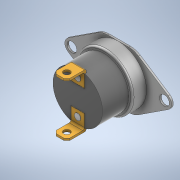
# Autodesk Inventor part: Bimetallschalter
Saved by Autodesk Inventor 2021 (Build 250183000, 183)
## iProperties
Created: 2021-04-29
Part Number: Bimetallschalter
Material: Generisch
Document SubType Name: Modeling
Designer: Sebastian Seewald
Density: 1 g/cm^3
Appearance: Vorgabe
Author: Sebastian Seewald
Autodesk Inventor part; units mm, degrees
ref_plane "YZ Plane" through (0, 0, 0) normal (1, 0, 0) x (0, 1, 0)
ref_plane "XZ Plane" through (0, 0, 0) normal (0, 1, 0) x (-1, 0, 0)
ref_plane "XY Plane" through (0, 0, 0) normal (0, 0, 1) x (1, 0, 0)
sketch "Skizze1" plane through (0, 0, 0) normal (0, 0, 1) x (1, 0, 0)
  line L0 (-3, 8) -> (3, 8)
  line L1 (5.7352, 7.1856) -> (14.1691, 1.6742)
  line L2 (14.1691, -1.6742) -> (5.7352, -7.1856)
  line L3 (3, -8) -> (-3, -8)
  line L4 (-5.7352, -7.1856) -> (-14.1691, -1.6742)
  line L5 (-14.1691, 1.6742) -> (-5.7352, 7.1856)
  arc A0 (14.1691, -1.6742) -> (14.1691, 1.6742) centre (13.075, 0) ccw
  arc A1 (-14.1691, 1.6742) -> (-14.1691, -1.6742) centre (-13.075, 0) ccw
  circle A2 centre (0, 0) radius 7
  circle A3 centre (-13.075, 0) radius 1.385
  circle A4 centre (13.075, 0) radius 1.385
  arc A5 (-3, 8) -> (-5.7352, 7.1856) centre (-3, 3) ccw
  arc A6 (5.7352, 7.1856) -> (3, 8) centre (3, 3) ccw
  arc A7 (3, -8) -> (5.7352, -7.1856) centre (3, -3) ccw
  arc A8 (-5.7352, -7.1856) -> (-3, -8) centre (-3, -3) ccw
  dimension "d0" = 16
  dimension "d1" = 8
  dimension "d3" = 2
  dimension "d4" = 14
  dimension "d5" = 30.15
  dimension "d7" = 2.77
  dimension "d8" = 2.77
  dimension "d9" = 13.075
  dimension "d10" = 13.075
  dimension "d11" = 5
  dimension "d12" = 6
  dimension "d13" = 6
  dimension "d14" = 3
  dimension "d15" = 3
  constraints: 12 end point, 12 point on circle, 12 tangent, 9 centre point, 4 equal radius, 3 coincident, 1 horizontal, 1 horizontal alignment, 1 parallel
  measures "d0" distance between parallel lines of L3 L0
  measures "d1" distance from line of point (0, 0) L0
  measures "d3" radius of A0
  measures "d4" diameter of A2
  measures "d7" diameter of A3
  measures "d8" diameter of A4
  measures "d9" distance of A1.centre point (0, 0)
  measures "d10" distance of A0.centre point (0, 0)
  measures "d11" radius of A5
  measures "d12" distance of L0.start L0.end
  measures "d13" distance of L3.start L3.end
  measures "d14" horizontal distance of point (0, 0) L0.start
  measures "d15" horizontal distance of point (0, 0) L3.end
extrude "Extrusion1" add sketch "Skizze1" along normal blind 0.5
sketch "Skizze2" plane through (0, 0, 0.5) normal (0, 0, 1) x (1, 0, 0)
  circle A0 centre (0, 0) radius 8
  circle A1 centre (0, 0) radius 7
  dimension "d18" = 16
  dimension "d19" = 14
  constraints: 2 centre point, 2 coincident
  measures "d18" diameter of A0
  measures "d19" diameter of A1
extrude "Extrusion2" add sketch "Skizze2" along normal blind 4
fillet "Rundung1" radius 0.5 1 edges at (-8, 0, 4.5)
sketch "Skizze3" plane through (0, 0, 0) normal (0, 0, -1) x (-1, 0, 0)
  circle A0 centre (0, 0) radius 7
  dimension "d23" = 14
  constraints: 1 centre point, 1 coincident
  measures "d23" diameter of A0
extrude "Extrusion3" add sketch "Skizze3" against normal blind 11.91
sketch "Skizze4" plane through (0, 0, 0) normal (0, 0, -1) x (-1, 0, 0)
  circle A0 centre (0, 3) radius 0.4
  point P0 (0, 0)
  dimension "d26" = 3
  dimension "d27" = 0.8
  constraints: 1 centre point, 1 vertical alignment
  measures "d26" distance of point (0, 0) A0.centre
  measures "d27" diameter of A0
extrude "Extrusion4" cut sketch "Skizze4" against normal blind 0.1
pattern_circular "Runde Anordnung1" count 3 over 360 about axis through (0, 0, -10) along (0, 0, 1) of "Extrusion4"
sketch "Skizze5" plane through (0, 0, 11.91) normal (0, 0, 1) x (1, 0, 0)
  line L0 (2, -9) -> (-2, -9)
  line L1 (-2, -9) -> (-2, -3)
  line L2 (-2, -3) -> (2, -3)
  line L3 (2, -3) -> (2, -9)
  line L4 (2, 3) -> (-2, 3)
  line L5 (-2, 3) -> (-2, 9)
  line L6 (-2, 9) -> (2, 9)
  line L7 (2, 9) -> (2, 3)
  line L8 (3, 8) -> (0, 8) projected
  line L9 (0, -8) -> (3, -8) projected
  point P0 (0, 0)
  dimension "d33" = 4
  dimension "d34" = 2
  dimension "d35" = 3
  dimension "d36" = 3
  dimension "d37" = 1
  dimension "d38" = 1
  constraints: 16 end point, 4 parallel, 2 horizontal, 2 perpendicular, 2 point on line
  measures "d33" distance between parallel lines of L3 L1
  measures "d34" distance from line of point (0, 0) L1
  measures "d35" distance from line of point (0, 0) L2
  measures "d36" distance from line of L4 point (0, 0)
  measures "d37" distance between parallel lines of L8 L6
  measures "d38" distance between parallel lines of L9 L0
extrude "Extrusion5" cut sketch "Skizze5" against normal blind 0.5
sketch "Skizze6" plane through (0, 0, 11.41) normal (0, 0, 1) x (1, 0, 0)
  line L0 (1.9, -7.6) -> (-1.9, -7.6)
  line L1 (-1.9, -7.6) -> (-1.9, -3.1)
  line L2 (-1.9, -3.1) -> (1.9, -3.1)
  line L3 (1.9, -3.1) -> (1.9, -7.6)
  line L4 (-2, -3) -> (2, -3) projected
  line L5 (1.9, 3.1) -> (-1.9, 3.1)
  line L6 (-1.9, 3.1) -> (-1.9, 7.6)
  line L7 (-1.9, 7.6) -> (1.9, 7.6)
  line L8 (1.9, 7.6) -> (1.9, 3.1)
  line L9 (2, 3) -> (-2, 3) projected
  point P0 (0, 0)
  dimension "d41" = 3.8
  dimension "d42" = 1.9
  dimension "d43" = 0.1
  dimension "d44" = 4.5
  dimension "d45" = 3.8
  dimension "d46" = 1.9
  dimension "d47" = 0.1
  dimension "d48" = 4.5
  constraints: 16 end point, 4 parallel, 2 horizontal, 2 perpendicular
  measures "d41" distance between parallel lines of L3 L1
  measures "d42" distance from line of point (0, 0) L3
  measures "d43" distance between parallel lines of L4 L2
  measures "d44" distance between parallel lines of L2 L0
  measures "d45" distance between parallel lines of L8 L6
  measures "d46" distance from line of point (0, 0) L8
  measures "d47" distance between parallel lines of L9 L5
  measures "d48" distance between parallel lines of L7 L5
extrude "Extrusion6" add sketch "Skizze6" along normal blind 0.5
sketch "Skizze7" plane through (0, 0, 11.91) normal (0, 0, 1) x (1, 0, 0)
  line L0 (1.9, 7.6) -> (-1.9, 7.6) projected
  line L1 (-1.9, 7.6) -> (-1.9, 3.1) projected
  line L2 (1.9, 7.6) -> (-1.9, 7.6)
  line L3 (-1.9, 7.6) -> (-1.9, 7)
  line L4 (-1.9, 7) -> (1.9, 7)
  line L5 (1.9, 7) -> (1.9, 7.6)
  line L6 (-1.9, -7.6) -> (1.9, -7.6) projected
  line L7 (-1.9, -3.1) -> (-1.9, -7.6) projected
  line L8 (1.9, -7.6) -> (-1.9, -7.6)
  line L9 (-1.9, -7.6) -> (-1.9, -7)
  line L10 (-1.9, -7) -> (1.9, -7)
  line L11 (1.9, -7) -> (1.9, -7.6)
  point P0 (0, 0)
  dimension "d51" = 0.6
  dimension "d52" = 0.6
  constraints: 16 end point, 4 parallel, 2 horizontal, 2 perpendicular, 2 point on line
  measures "d51" distance between parallel lines of L0 L4
  measures "d52" distance between parallel lines of L6 L10
extrude "Extrusion7" add sketch "Skizze7" along normal blind 5
chamfer "Fase1" distance 0.8 angle 45 4 edges at (-1.9, 7.3, 16.91) (1.9, 7.3, 16.91) (-1.9, -7.3, 16.91) (1.9, -7.3, 16.91)
fillet "Rundung2" radius 0.5 4 edges at (0, 7.6, 11.41) (0, -7.6, 11.41) (0, -7, 11.91) (0, 7, 11.91)
sketch "Skizze8" plane through (-1.1, 7.6, 16.91) normal (0, 1, 0) x (1, 0, 0)
  circle A0 centre (1.1, 1.9) radius 0.9
  line L0 (2.2, 0) -> (0, 0) projected
  point P0 (1.1, 16.91)
  dimension "d59" = 1.8
  dimension "d60" = 1.9
  constraints: 1 centre point
  measures "d59" diameter of A0
  measures "d60" distance from line of L0 A0.centre
extrude "Extrusion8" cut sketch "Skizze8" against normal blind 20
sketch "Skizze9" plane through (0, 0, 11.91) normal (0, 0, 1) x (1, 0, 0)
  circle A0 centre (0, 4.8) radius 0.9
  circle A1 centre (0, -4.8) radius 0.9
  point P0 (0, 0)
  dimension "d63" = 1.8
  dimension "d64" = 1.8
  dimension "d65" = 4.8
  dimension "d66" = 4.8
  constraints: 2 centre point, 2 vertical alignment
  measures "d63" diameter of A0
  measures "d64" diameter of A1
  measures "d65" distance of point (0, 0) A1.centre
  measures "d66" distance of point (0, 0) A0.centre
extrude "Extrusion9" add sketch "Skizze9" along normal blind 0.1
